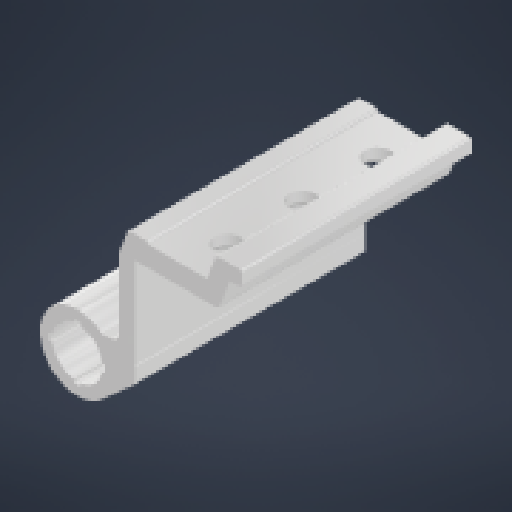
# Autodesk Inventor part: HIN-61 BISAGRA (P2)
Saved by Autodesk Inventor 2025 (Build 290162000, 162)
## iProperties
Created: 2026-02-04
Part Number: HIN-61 BISAGRA (P2)
Material: Aluminio
Document SubType Name: Modeling
Designer: ROLANDO
Density: 2.7 g/cm^3
Appearance: Satinado
Author: ROLANDO
Autodesk Inventor part; units mm, degrees
ref_plane "YZ Plane" through (0, 0, 0) normal (1, 0, 0) x (0, 1, 0)
ref_plane "XZ Plane" through (0, 0, 0) normal (0, 1, 0) x (-1, 0, 0)
ref_plane "XY Plane" through (0, 0, 0) normal (0, 0, 1) x (1, 0, 0)
sketch "Boceto1" plane through (0, 0, 0) normal (0, 0, 1) x (1, 0, 0)
  arc A0 (4.8153, 5.75) -> (5.0185, -5.5736) centre (0, 0) ccw
  line L0 (0, 12.1119) -> (0, -11.4197) construction
  line L1 (-11.1817, 0) -> (12.1806, 0) construction
  line L2 (4.9434, 0.75) -> (5.5, 0.75)
  line L3 (4.9434, -0.75) -> (5.5, -0.75)
  line L4 (5.5, -0.75) -> (5.5, 0.75)
  line L5 (-0.75, 4.9434) -> (-0.75, 5.5)
  line L6 (0.75, 5.5) -> (-0.75, 5.5)
  line L7 (0.75, 4.9434) -> (0.75, 5.5)
  line L8 (-4.9434, -0.75) -> (-5.5, -0.75)
  line L9 (-5.5, 0.75) -> (-5.5, -0.75)
  line L10 (-4.9434, 0.75) -> (-5.5, 0.75)
  line L11 (0.75, -4.9434) -> (0.75, -5.5)
  line L12 (-0.75, -5.5) -> (0.75, -5.5)
  line L13 (-0.75, -4.9434) -> (-0.75, -5.5)
  arc A1 (-0.75, 4.9434) -> (-4.9434, 0.75) centre (0, 0) ccw
  arc A2 (-4.9434, -0.75) -> (-0.75, -4.9434) centre (0, 0) ccw
  arc A3 (0.75, -4.9434) -> (4.9434, -0.75) centre (0, 0) ccw
  arc A4 (4.9434, 0.75) -> (0.75, 4.9434) centre (0, 0) ccw
  circle A5 centre (0, 0) radius 5 construction
  line L14 (-11.772, 7.5) -> (14.517, 7.5) construction
  line L15 (-11.772, -7.5) -> (14.517, -7.5) construction
  line L16 (4.8153, 5.75) -> (6.5, 5.75)
  line L17 (8.5, 7.75) -> (8.5, 21.6618)
  line L18 (14.1379, 25.75) -> (25.6337, 25.75)
  line L19 (11.5, 21.75) -> (11.5, 3.4624)
  arc A6 (6.5, 5.75) -> (8.5, 7.75) centre (6.5, 7.75) ccw
  line L20 (5.0185, -5.5736) -> (11.5, 0.2624)
  line L21 (11.5, 21.75) -> (27.5524, 21.75)
  line L22 (28.4921, 22.408) -> (30.4, 27.65)
  line L23 (30.4, 27.65) -> (32.4, 27.65)
  line L24 (32.9, 28.15) -> (32.9, 30.15)
  line L25 (32.4, 30.65) -> (28.1174, 30.65)
  line L26 (27.6475, 30.321) -> (26.1036, 26.079)
  line L27 (14.1379, 25.75) -> (14.1379, 25.75)
  line L28 (13.6379, 26.25) -> (10.488, 26.25)
  line L29 (10.0181, 25.921) -> (8.5302, 21.8328)
  line L30 (11.5, 0.2624) -> (11.5, 3.2624)
  line L31 (12.5556, 3.3624) -> (11.7894, 3.3624) construction
  line L32 (11.5, 3.4624) -> (11.4, 3.3624)
  line L33 (11.5, 3.2624) -> (11.4, 3.3624)
  arc A7 (32.4, 27.65) -> (32.9, 28.15) centre (32.4, 28.15) ccw
  arc A8 (32.9, 30.15) -> (32.4, 30.65) centre (32.4, 30.15) ccw
  arc A9 (28.1174, 30.65) -> (27.6475, 30.321) centre (28.1174, 30.15) ccw
  arc A10 (14.1379, 25.75) -> (13.6379, 26.25) centre (13.6379, 25.75) ccw
  arc A11 (10.488, 26.25) -> (10.0181, 25.921) centre (10.488, 25.75) ccw
  arc A12 (25.6337, 25.75) -> (26.1036, 26.079) centre (25.6337, 26.25) ccw
  arc A13 (27.5524, 21.75) -> (28.4921, 22.408) centre (27.5524, 22.75) ccw
  arc A14 (8.5302, 21.8328) -> (8.5, 21.6618) centre (9, 21.6618) ccw
  point P0 (25.9838, 25.75)
  point P1 (8.5, 21.75)
  point P2 (28.2526, 21.75)
  point P3 (32.9, 27.65)
  point P4 (32.9, 30.65)
  point P5 (27.7673, 30.65)
  point P6 (14.1379, 26.25)
  point P7 (10.1379, 26.25)
  dimension "d0" = 15
  dimension "d4" = 0.75
  dimension "d6" = 1.5
  dimension "d11" = 360
  dimension "d13" = 10
  dimension "d14" = 0.5
  dimension "d15" = 5
  dimension "d16" = 1.75
  dimension "d22" = 3
  dimension "d27" = 20
  dimension "d49" = 2
  dimension "d89" = 4
  dimension "d90" = 3
  dimension "d91" = 3.5
  dimension "d92" = 4
  dimension "d93" = 0.5
  dimension "d96" = 2.5
  dimension "d97" = 4.5
  dimension "d98" = 3
  dimension "d100" = 48
  dimension "d101" = 0.2
  dimension "d102" = 0.1
  dimension "d106" = 0.1
  dimension "d108" = 70
  dimension "d111" = 24.4
  dimension "d113" = 19
  dimension "d118" = 70
  dimension "d123" = 0.5
  dimension "d124" = 1
  dimension "d125" = 0.5
  dimension "d155" = 8.9
  dimension "d156" = 38.15
  constraints: 68 end point, 28 point on circle, 21 tangent, 20 point on line, 15 centre point, 9 horizontal, 6 perpendicular, 5 equal radius, 4 vertical, 3 coincident, 1 parallel, 29 other
  measures "d0" diameter of A0
  measures "d4" distance between parallel lines of L1 L3
  measures "d6" distance between parallel lines of L3 L2
  measures "d13" diameter of A5
  measures "d14" distance edge to line of A5 L6
  measures "d15" radius of A4
  measures "d16" distance between parallel lines of L14 L16
  measures "d22" distance between parallel lines of L17 L19
  measures "d27" distance between parallel lines of L18 L16
  measures "d49" radius of A6
  measures "d89" distance between parallel lines of L21 L18
  measures "d90" distance between parallel lines of L25 L23
  measures "d91" distance between parallel lines of L26 L22
  measures "d92" distance of point (14.138, 26.25) point (10.138, 26.25)
  measures "d93" distance of L18.start point (14.138, 26.25)
  measures "d96" distance of L22.end point (32.9, 27.65)
  measures "d97" vertical distance of point (10.138, 26.25) point (8.5, 21.75)
  measures "d98" distance of L20.end L30.end
  measures "d100" angle of L30 L20
  measures "d101" distance of L30.end L19.end
  measures "d102" distance from line of L19.end L31
  measures "d106" horizontal distance of L32.end L19.end
  measures "d108" angle of L21 L29
  measures "d111" distance between parallel lines of L24 L17
  measures "d118" angle of L21 L22
  measures "d123" radius of A7
  measures "d124" radius of A13
  measures "d125" radius of A14
  measures "d155" distance between parallel lines of L25 L21
  measures "d156" distance between parallel lines of L15 L25
extrude "Extrusión1" add sketch "Boceto1" against normal blind 46
sketch "Boceto2" plane through (11.5, 21.75, 0) normal (0, -1, 0) x (1, 0, 0)
  line L0 (10.4674, 0.9421) -> (10.4674, -47.0057) construction
  line L1 (16.0524, 0) -> (16.0524, -46) projected
  line L2 (0, 0) -> (0, -46) projected
  line L3 (-0.8036, -23) -> (23.8698, -23) construction
  line L4 (0, 0) -> (16.0524, 0) projected
  line L5 (16.0524, -46) -> (0, -46) projected
  circle A0 centre (10.4674, -23) radius 2.5
  circle A1 centre (10.4674, -23) radius 4.5
  circle A2 centre (10.4674, -38) radius 2.5
  circle A3 centre (10.4674, -38) radius 4.5
  circle A4 centre (10.4674, -8) radius 2.5
  circle A5 centre (10.4674, -8) radius 4.5
  point P0 (-11.5, 0)
  dimension "d134" = 5.585
  dimension "d136" = 23
  dimension "d137" = 23
  dimension "d138" = 5
  dimension "d139" = 9
  dimension "d140" = 2
  dimension "d143" = 15
  constraints: 6 centre point, 4 end point, 3 coincident, 2 point on line, 2 vertical, 1 horizontal, 8 other
  measures "d134" distance between parallel lines of L1 L0
  measures "d136" distance between parallel lines of L4 L3
  measures "d137" distance between parallel lines of L5 L3
  measures "d138" diameter of A0
  measures "d139" diameter of A1
  measures "d140" radial gap between concentric circles of A1 A0
  measures "d143" distance of A0.centre A2.centre
hole "Agujero2" at (21.9674, 21.75, -8) at (21.9674, 21.75, -23) at (21.9674, 21.75, -38) direction (0, 1, 0) diameter 5 end through all countersink diameter 9 countersink angle 90
